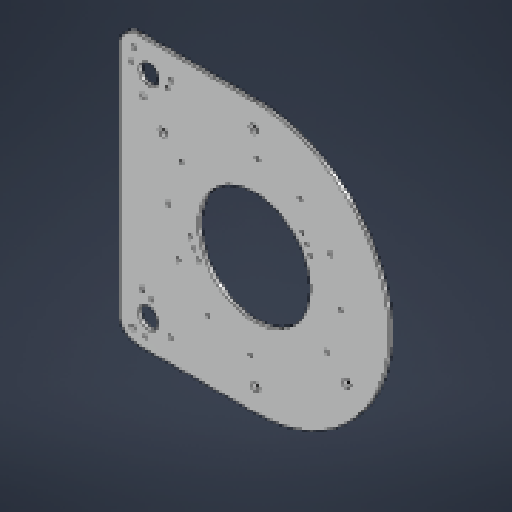
# Autodesk Inventor part: PLATE,SHOOTER,MOUNT
Saved by Autodesk Inventor 2026 (Build 300175000, 175)
## iProperties
Created: 2026-02-09
Part Number: PLATE,SHOOTER,MOUNT
Material: Aluminum 6061
Document SubType Name: Sheet Metal
Designer: littl
Density: 2.7 g/cm^3
Sheet Metal Rule: Default
Appearance: Aluminum - Flat
Mass: 1386.25 g
Surface Area: 2270.1 cm^2
Volume: 513.425 cm^3
Author: littl
Autodesk Inventor part; units mm, degrees
ref_plane "YZ Plane" through (0, 0, 0) normal (1, 0, 0) x (0, 1, 0)
ref_plane "XZ Plane" through (0, 0, 0) normal (0, 1, 0) x (-1, 0, 0)
ref_plane "XY Plane" through (0, 0, 0) normal (0, 0, 1) x (1, 0, 0)
sketch "Sketch1" plane through (0, 0, 0) normal (0, 0, 1) x (1, 0, 0)
  line L0 (-190.5, -190.5) -> (190.5, -190.5)
  line L1 (190.5, -190.5) -> (190.5, 190.5)
  line L2 (190.5, 190.5) -> (-190.5, 190.5)
  line L3 (-190.5, 190.5) -> (-190.5, -190.5)
  line L4 (-190.5, -190.5) -> (190.5, 190.5) construction
  line L5 (190.5, -190.5) -> (-190.5, 190.5) construction
  circle A0 centre (0, 0) radius 79.375
  line L6 (130.599, -90.0738) -> (-0.5713, 156.6217) construction
  line L7 (-0.5713, 156.6217) -> (-129.5258, 88.0554) construction
  line L8 (-129.5258, 88.0554) -> (1.6445, -158.6401) construction
  line L9 (1.6445, -158.6401) -> (130.599, -90.0738) construction
  line L10 (130.599, -90.0738) -> (-129.5258, 88.0554) construction
  line L11 (-0.5713, 156.6217) -> (1.6445, -158.6401) construction
  line L12 (1.6445, -158.6401) -> (-64.4772, -34.2832) construction
  line L13 (-64.4772, -34.2832) -> (-12.5828, -6.6904) construction
  line L14 (-65.0486, 122.3386) -> (66.1218, -124.357) construction
  line L15 (-91.2837, -21.0636) -> (-75.8652, -12.8655) construction
  line L16 (-91.2837, -21.0636) -> (-85.3214, -32.2771) construction
  line L17 (-85.3214, -32.2771) -> (-79.3591, -43.4905) construction
  line L18 (68.5077, 63.899) -> (53.0893, 55.7008) construction
  line L19 (68.5077, 63.899) -> (74.47, 52.6855) construction
  line L20 (74.47, 52.6855) -> (80.4323, 41.4721) construction
  arc A1 (0, -190.5) -> (190.5, 0) centre (0, 0) ccw
  arc A2 (190.5, 0) -> (0, 190.5) centre (0, 0) ccw
  point P0 (0.5366, -1.0092)
  point P1 (152.4, 190.5)
  point P2 (-17.6976, -190.5)
  dimension "d0" = 381
  dimension "d1" = 158.75
  dimension "d2" = 279.4
  dimension "d3" = 146.05
  dimension "d4" = 28
  dimension "d5" = 140.843
  dimension "d6" = 114.3
  dimension "d7" = 17.4625
  dimension "d8" = 12.7
  dimension "d9" = 114.3
  dimension "d11" = 17.4625
  dimension "d12" = 12.7
  constraints: 42 end point, 9 midpoint, 7 coincident, 7 point on line, 6 parallel, 5 perpendicular, 4 point on circle, 3 centre point, 3 equal length, 2 collinear, 1 horizontal
  measures "d0" distance of L2.end L1.end
  measures "d1" diameter of A0
  measures "d2" distance of L6.start L6.end
  measures "d3" distance of L6.end L7.end
  measures "d4" angle of L3 L8
  measures "d5" distance of L8.end L12.end
  measures "d6" distance between parallel lines of L7 L15
  measures "d7" distance of L15.start L15.end
  measures "d8" distance of L15.start L16.end
  measures "d9" distance between parallel lines of L7 L18
  measures "d11" distance of L18.start L18.end
  measures "d12" distance of L19.end L20.end
extrude "Plate1" add sketch "Sketch1" along normal blind 4.7752 contours L3 L2 A2 A1 L0
hole "Hole1" at (-91.2837, -21.0636, 0) at (-85.3214, -32.2771, 0) at (-79.3591, -43.4905, 0) at (68.5077, 63.899, 0) at (74.47, 52.6855, 0) at (80.4323, 41.4721, 0) direction (0, 0, 1) diameter 4.9784 end through all clearance for "Flat Head Machine Screw (82)" size "#10" standard "Ansi Unified Screw Threads"
fillet "Corner Round1" radius 25.4 2 edges at (-190.5, 190.5, 2.3876) (-190.5, -190.5, 2.3876)
sketch "Sketch7" plane through (0, 0, 4.7752) normal (0, 0, 1) x (1, 0, 0)
  line L0 (0, 0) -> (-126.9226, 4.4322) construction
  line L1 (0, 266.7) -> (0, -266.7) projected
  circle A0 centre (-79.3591, -43.4905) radius 2.4892 projected
  circle A1 centre (80.4323, 41.4721) radius 2.4892 projected
  line L2 (59.6229, -112.1343) -> (0, 0) construction
  circle A2 centre (-91.2837, -21.0636) radius 2.4892 projected
  circle A3 centre (68.5077, 63.899) radius 2.4892 projected
  line L3 (-91.2837, -21.0636) -> (-79.3591, -43.4905) construction
  line L4 (68.5077, 63.899) -> (80.4323, 41.4721) construction
  point P0 (-112.1343, -59.6229)
  point P1 (-67.2997, -107.7021)
  point P2 (-4.4322, -126.9226)
  point P3 (107.7021, -67.2997)
  point P4 (126.9226, -4.4322)
  point P5 (112.1343, 59.6229)
  point P6 (67.2997, 107.7021)
  point P7 (4.4322, 126.9226)
  point P8 (-59.6229, 112.1343)
  point P9 (-107.7021, 67.2997)
  dimension "d94" = 127
  dimension "d98" = 360
  constraints: 8 end point, 1 parallel, 13 other
  measures "d94" distance of L0.start L0.end
hole "Hole6" at (-126.9226, 4.4322, 4.7752) at (-67.2997, -107.7021, 4.7752) at (-4.4322, -126.9226, 4.7752) at (107.7021, -67.2997, 4.7752) at (126.9226, -4.4322, 4.7752) at (4.4322, 126.9226, 4.7752) at (67.2997, 107.7021, 4.7752) at (-107.7021, 67.2997, 4.7752) direction (0, 0, -1) diameter 4.9784 end through all clearance for "Flat Head Machine Screw (82)" size "#10" standard "Ansi Unified Screw Threads"
sketch "Sketch8" plane through (0, 0, 4.7752) normal (0, 0, 1) x (1, 0, 0)
  circle A0 centre (0, 0) radius 190.5 construction
  arc A1 (-165.1, 190.5) -> (-190.5, 165.1) centre (-165.1, 165.1) ccw projected
  line L0 (-165.1, 165.1) -> (0, 0) construction
  arc A2 (-190.5, -165.1) -> (-165.1, -190.5) centre (-165.1, -165.1) ccw projected
  line L1 (0, 0) -> (-165.1, -165.1) construction
  line L2 (-149.9703, -149.9703) -> (-172.4209, -172.4209) construction
  line L3 (-149.0723, 149.0723) -> (-171.5229, 171.5229) construction
  line L4 (-149.0723, 149.0723) -> (-123.9351, 145.4275) construction
  line L5 (-149.0723, 149.0723) -> (-128.558, 149.0723) construction
  line L6 (-149.9703, -149.9703) -> (-145.5596, -124.9562) construction
  line L7 (-149.9703, -149.9703) -> (-130.8542, -149.9703)
  point P0 (-119.3021, -158.1878)
  point P1 (-158.1878, -119.3021)
  point P2 (-157.2898, 118.4041)
  point P3 (-118.4041, 157.2898)
  point P4 (-174.2094, 152.717)
  point P5 (-154.3809, -174.9844)
  dimension "d107" = 381
  dimension "d108" = 212.09
  dimension "d109" = 210.82
  dimension "d110" = 31.75
  dimension "d113" = 360
  dimension "d115" = 31.75
  dimension "d118" = 360
  dimension "d134" = 25.4
  dimension "d137" = 360
  dimension "d139" = 8.25
  dimension "d149" = 360
  dimension "d151" = 25.4
  dimension "d153" = 80
  constraints: 16 end point, 2 coincident, 2 collinear, 2 horizontal, 2 point on line, 1 centre point, 1 perpendicular, 14 other
  measures "d107" diameter of A0
  measures "d108" distance of point (0, 0) L2.start
  measures "d109" distance of point (0, 0) L3.start
  measures "d110" distance of L2.start L2.end
  measures "d115" distance of L3.start L3.end
  measures "d134" distance of L3.start L4.end
  measures "d139" angle of L4 L5
  measures "d151" distance of L2.start L6.end
  measures "d153" angle of L7 L6
hole "Hole7" at (-172.4209, -172.4209, 4.7752) at (-119.3021, -158.1878, 4.7752) at (-158.1878, -119.3021, 4.7752) at (-171.5229, 171.5229, 4.7752) at (-157.2898, 118.4041, 4.7752) at (-118.4041, 157.2898, 4.7752) direction (0, 0, -1) diameter 6.5278 depth 4.7752 tip angle 118 clearance for "Flat Head Machine Screw (82)" size "1/4" standard "Ansi Unified Screw Threads"
hole "Hole8" at (-149.0723, 149.0723, 4.7752) at (-149.9703, -149.9703, 4.7752) direction (0, 0, -1) diameter 28.575 depth 4.7752 tip angle 118
hole "Hole9" at (-123.9351, 145.4275, 4.7752) at (-174.2094, 152.717, 4.7752) at (-154.3809, -174.9844, 4.7752) at (-145.5596, -124.9562, 4.7752) direction (0, 0, -1) diameter 4.9784 end through all clearance for "Flat Head Machine Screw (82)" size "#10" standard "Ansi Unified Screw Threads"
sketch "Sketch9" plane through (0, 0, 4.7752) normal (0, 0, 1) x (1, 0, 0)
  point P0 (0, 0)
  point P1 (1.6445, -158.6401)
  point P2 (130.599, -90.0738)
  point P3 (-0.5713, 156.6217)
  point P4 (-129.5258, 88.0554)
  point P5 (-129.5258, 88.0554)
  point P6 (1.6445, -158.6401)
  point P7 (130.599, -90.0738)
  point P8 (-0.5713, 156.6217)
  constraints: 4 coincident
hole "Hole11" at (-0.5713, 156.6217, 4.7752) at (-129.5258, 88.0554, 4.7752) at (1.6445, -158.6401, 4.7752) at (130.599, -90.0738, 4.7752) direction (0, 0, -1) diameter 4.9784 end through all countersink diameter 10.668 countersink angle 82 clearance for "Flat Head Machine Screw (82)" size "#10" standard "Ansi Unified Screw Threads"
equation "\"d11\" = d7"
equation "\"d19\" = Thickness"
equation "\"d105\" = Thickness"
equation "\"d125\" = Thickness"
equation "\"d132\" = Thickness"
equation "\"d13\" = Thickness"
equation "\"BendRadius\" = Thickness"
equation "\"BendReliefWidth\" = Thickness"
equation "\"BendReliefDepth\" = 0.5 * Thickness"
equation "\"CornerReliefSize\" = 4 * Thickness"
equation "\"MinimumRemnant\" = 2 * Thickness"
equation "\"TransitionRadius\" = BendRadius"
equation "\"JacobiRadiusSize\" = BendRadius"
equation "\"GapSize\" = Thickness"
equation "\"Thickness\" = 4.7752"
body "Solid1"
